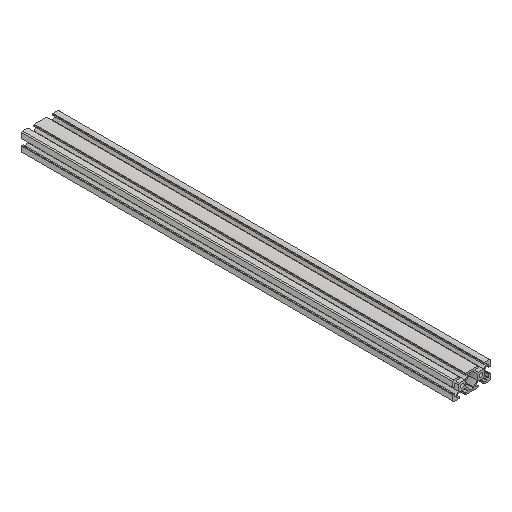
# Autodesk Inventor part: COTS_GENERIC_20x40mm_alu_extrusion_460mm
Saved by Autodesk Inventor 2026.1 (Build 301233000, 233)
## iProperties
Created: 2017-05-24
Part Number: COTS_GENERIC_20x40mm_alu_extrusion_460mm
Material: Ogólny
Document SubType Name: Modeling
Designer: Andrzej
Density: 1 g/cm^3
Appearance: Aluminium - polerowane
Mass: 147.48 g
Surface Area: 1432.83 cm^2
Volume: 147.48 cm^3
Author: Andrzej
Autodesk Inventor part; units mm, degrees
ref_plane "YZ Plane" through (0, 0, 0) normal (1, 0, 0) x (0, 1, 0)
ref_plane "XZ Plane" through (0, 0, 0) normal (0, 1, 0) x (-1, 0, 0)
ref_plane "XY Plane" through (0, 0, 0) normal (0, 0, 1) x (1, 0, 0)
sketch "Szkic1" plane through (0, 0, 0) normal (1, 0, 0) x (0, 1, 0)
  line L0 (23.5169, -0.1319) -> (-36.4831, -0.1319)
  line L1 (-2.0853, 36.7703) -> (-2.0853, -38.5298)
  line L2 (17.9147, 2.8681) -> (15.9147, 2.8681)
  line L3 (17.9147, 2.8681) -> (17.9147, 9.8681)
  line L4 (17.9147, 9.8681) -> (10.9147, 9.8681)
  line L5 (10.9147, 9.8681) -> (10.9147, 7.8681)
  line L6 (15.9147, 2.8681) -> (15.9147, 5.8681)
  line L7 (10.9147, 7.8681) -> (13.9147, 7.8681)
  line L8 (13.9147, 7.8681) -> (13.9147, 6.8681)
  line L9 (15.9147, 5.8681) -> (14.9147, 5.8681)
  line L10 (11.9147, -0.1319) -> (11.9147, 2.8681)
  line L11 (10.9147, 3.8681) -> (4.9147, 3.8681)
  line L12 (3.9147, 2.8681) -> (3.9147, -0.1319)
  line L13 (4.9147, 7.8681) -> (4.9147, 9.8681)
  line L14 (4.9147, 9.8681) -> (-2.0853, 9.8681)
  line L15 (4.9147, 7.8681) -> (1.9147, 7.8681)
  line L16 (1.9147, 7.8681) -> (1.9147, 6.8681)
  line L17 (-0.0853, 7.8681) -> (-0.0853, 6.8681)
  line L18 (-0.0853, 7.8681) -> (-2.0853, 7.8681)
  line L19 (1.9147, 6.8681) -> (4.9147, 3.8681)
  line L20 (1.9147, 6.8681) -> (8.4857, 6.8681) construction
  line L21 (-0.0853, 6.8681) -> (3.9147, 2.8681)
  line L22 (-0.0853, 6.8681) -> (7.9037, 6.8681) construction
  line L23 (14.9147, 5.8681) -> (11.9147, 2.8681)
  line L24 (14.9147, 5.8681) -> (20.5717, 5.8681) construction
  line L25 (13.9147, 6.8681) -> (10.9147, 3.8681)
  line L26 (13.9147, 6.8681) -> (19.5717, 6.8681) construction
  line L27 (17.9147, -3.1319) -> (15.9147, -3.1319)
  line L28 (17.9147, -3.1319) -> (17.9147, -10.1319)
  line L29 (17.9147, -10.1319) -> (10.9147, -10.1319)
  line L30 (10.9147, -10.1319) -> (10.9147, -8.1319)
  line L31 (15.9147, -3.1319) -> (15.9147, -6.1319)
  line L32 (10.9147, -8.1319) -> (13.9147, -8.1319)
  line L33 (13.9147, -8.1319) -> (13.9147, -7.1319)
  line L34 (15.9147, -6.1319) -> (14.9147, -6.1319)
  line L35 (11.9147, -0.1319) -> (11.9147, -3.1319)
  line L36 (10.9147, -4.1319) -> (4.9147, -4.1319)
  line L37 (3.9147, -3.1319) -> (3.9147, -0.1319)
  line L38 (4.9147, -8.1319) -> (4.9147, -10.1319)
  line L39 (4.9147, -10.1319) -> (-2.0853, -10.1319)
  line L40 (4.9147, -8.1319) -> (1.9147, -8.1319)
  line L41 (1.9147, -8.1319) -> (1.9147, -7.1319)
  line L42 (-0.0853, -8.1319) -> (-0.0853, -7.1319)
  line L43 (-0.0853, -8.1319) -> (-2.0853, -8.1319)
  line L44 (1.9147, -7.1319) -> (4.9147, -4.1319)
  line L45 (1.9147, -7.1319) -> (8.4857, -7.1319) construction
  line L46 (-0.0853, -7.1319) -> (3.9147, -3.1319)
  line L47 (-0.0853, -7.1319) -> (7.9037, -7.1319) construction
  line L48 (14.9147, -6.1319) -> (11.9147, -3.1319)
  line L49 (13.9147, -7.1319) -> (10.9147, -4.1319)
  line L50 (13.9147, -7.1319) -> (19.5717, -7.1319) construction
  line L51 (-22.0853, 2.8681) -> (-20.0853, 2.8681)
  line L52 (-22.0853, 2.8681) -> (-22.0853, 9.8681)
  line L53 (-22.0853, 9.8681) -> (-15.0853, 9.8681)
  line L54 (-15.0853, 9.8681) -> (-15.0853, 7.8681)
  line L55 (-20.0853, 2.8681) -> (-20.0853, 5.8681)
  line L56 (-15.0853, 7.8681) -> (-18.0853, 7.8681)
  line L57 (-18.0853, 7.8681) -> (-18.0853, 6.8681)
  line L58 (-20.0853, 5.8681) -> (-19.0853, 5.8681)
  line L59 (-16.0853, -0.1319) -> (-16.0853, 2.8681)
  line L60 (-15.0853, 3.8681) -> (-9.0853, 3.8681)
  line L61 (-8.0853, 2.8681) -> (-8.0853, -0.1319)
  line L62 (-9.0853, 7.8681) -> (-9.0853, 9.8681)
  line L63 (-9.0853, 9.8681) -> (-2.0853, 9.8681)
  line L64 (-9.0853, 7.8681) -> (-6.0853, 7.8681)
  line L65 (-6.0853, 7.8681) -> (-6.0853, 6.8681)
  line L66 (-4.0853, 7.8681) -> (-4.0853, 6.8681)
  line L67 (-4.0853, 7.8681) -> (-2.0853, 7.8681)
  line L68 (-6.0853, 6.8681) -> (-9.0853, 3.8681)
  line L69 (-6.0853, 6.8681) -> (-12.6563, 6.8681) construction
  line L70 (-4.0853, 6.8681) -> (-8.0853, 2.8681)
  line L71 (-4.0853, 6.8681) -> (-12.0743, 6.8681) construction
  line L72 (-19.0853, 5.8681) -> (-16.0853, 2.8681)
  line L73 (-19.0853, 5.8681) -> (-24.7423, 5.8681) construction
  line L74 (-18.0853, 6.8681) -> (-15.0853, 3.8681)
  line L75 (-18.0853, 6.8681) -> (-23.7423, 6.8681) construction
  line L76 (-6.0853, -7.1319) -> (-12.6563, -7.1319) construction
  line L77 (-6.0853, -7.1319) -> (-9.0853, -4.1319)
  line L78 (-4.0853, -7.1319) -> (-12.0743, -7.1319) construction
  line L79 (-4.0853, -8.1319) -> (-4.0853, -7.1319)
  line L80 (-4.0853, -7.1319) -> (-8.0853, -3.1319)
  line L81 (-6.0853, -8.1319) -> (-6.0853, -7.1319)
  line L82 (-9.0853, -8.1319) -> (-6.0853, -8.1319)
  line L83 (-4.0853, -8.1319) -> (-2.0853, -8.1319)
  line L84 (-15.0853, -10.1319) -> (-15.0853, -8.1319)
  line L85 (-9.0853, -10.1319) -> (-2.0853, -10.1319)
  line L86 (-9.0853, -8.1319) -> (-9.0853, -10.1319)
  line L87 (-15.0853, -4.1319) -> (-9.0853, -4.1319)
  line L88 (-8.0853, -3.1319) -> (-8.0853, -0.1319)
  line L89 (-22.0853, -3.1319) -> (-20.0853, -3.1319)
  line L90 (-22.0853, -3.1319) -> (-22.0853, -10.1319)
  line L91 (-22.0853, -10.1319) -> (-15.0853, -10.1319)
  line L92 (-20.0853, -3.1319) -> (-20.0853, -6.1319)
  line L93 (-15.0853, -8.1319) -> (-18.0853, -8.1319)
  line L94 (-18.0853, -8.1319) -> (-18.0853, -7.1319)
  line L95 (-20.0853, -6.1319) -> (-19.0853, -6.1319)
  line L96 (-18.0853, -7.1319) -> (-15.0853, -4.1319)
  line L97 (-19.0853, -6.1319) -> (-16.0853, -3.1319)
  line L98 (-18.0853, -7.1319) -> (-23.7423, -7.1319) construction
  line L99 (-16.0853, -0.1319) -> (-16.0853, -3.1319)
  point P0 (0, 0)
  point P1 (0, -0.2637)
  point P2 (-4.1707, 0)
  point P3 (-4.1707, -0.2637)
  dimension "d1" = 2
  dimension "d2" = 3
  dimension "d3" = 7
  dimension "d4" = 7
  dimension "d5" = 2
  dimension "d6" = 3
  dimension "d7" = 3
  dimension "d8" = 1
  dimension "d9" = 1
  dimension "d12" = 6
  dimension "d13" = 2
  dimension "d14" = 7
  dimension "d15" = 6
  dimension "d16" = 3
  dimension "d17" = 1
  dimension "d18" = 1
  dimension "d19" = 2
  dimension "d20" = 8
  dimension "d22" = 45
  dimension "d24" = 45
  dimension "d26" = 135
  dimension "d28" = 135
  dimension "d29" = 6
  dimension "d30" = 4
  dimension "d31" = 3
  dimension "d32" = 3
  dimension "d33" = 8
  dimension "d34" = 1
  constraints: 200 end point, 74 symmetric about line, 9 horizontal, 9 vertical, 5 perpendicular, 4 point on line
  measures "d1" distance of L2.start L2.end
  measures "d2" distance between parallel lines of L0 L2
  measures "d3" distance of L2.start L3.end
  measures "d4" distance of L3.end L4.end
  measures "d5" distance of L4.end L5.end
  measures "d6" distance of L2.end L6.end
  measures "d7" distance of L5.end L7.end
  measures "d8" distance of L7.end L8.end
  measures "d9" distance of L6.end L9.end
  measures "d12" distance between parallel lines of L3 L10
  measures "d13" distance of L13.start L13.end
  measures "d14" distance of L13.end L14.end
  measures "d15" distance between parallel lines of L5 L13
  measures "d16" distance of L13.start L15.end
  measures "d17" distance of L15.end L16.end
  measures "d18" distance of L17.start L17.end
  measures "d19" distance between parallel lines of L16 L17
  measures "d20" distance between parallel lines of L0 L15
  measures "d22" angle of L19 L20
  measures "d24" angle of L21 L22
  measures "d26" angle of L23 L24
  measures "d28" angle of L25 L26
  measures "d29" distance of L11.start L11.end
  measures "d30" distance between parallel lines of L0 L11
  measures "d31" distance of L10.start L10.end
  measures "d32" distance of L12.start L12.end
  measures "d33" distance between parallel lines of L10 L12
  measures "d34" distance from line of L10 L11.start
extrude "Wyciągnięcie proste1" add sketch "Szkic1" along normal blind 460 contours L35 L48 L34 L31 L27 L28 L29 L30 L32 L33 L49 L36 L44 L41 L40 L38 L39 L1 L43 L42 L46 L37 L0 | L0 L12 L21 L17 L18 L1 L14 L13 L15 L16 L19 L11 L25 L8 L7 L5 L4 L3 L2 L6 L9 L23 L10 | L88 L80 L79 L83 L1 L85 L86 L82 L81 L77 L87 L96 L94 L93 L84 L91 L90 L89 L92 L95 L97 L99 L0 | L0 L59 L72 L58 L55 L51 L52 L53 L54 L56 L57 L74 L60 L68 L65 L64 L62 L63 L1 L67 L66 L70 L61
sketch "Szkic2" plane through (460, 0, 0) normal (1, 0, 0) x (0, 0, -1)
  line L0 (-7.8681, -4.0853) -> (-7.8681, -0.0853) projected
  line L1 (-7.8681, -0.0853) -> (-6.8681, -0.0853) projected
  line L2 (-6.8681, -0.0853) -> (-2.8681, 3.9147) projected
  line L3 (-2.8681, 3.9147) -> (3.1319, 3.9147) projected
  line L4 (3.1319, 3.9147) -> (7.1319, -0.0853) projected
  line L5 (7.1319, -0.0853) -> (8.1319, -0.0853) projected
  line L6 (8.1319, -0.0853) -> (8.1319, -4.0853) projected
  line L7 (8.1319, -4.0853) -> (7.1319, -4.0853) projected
  line L8 (7.1319, -4.0853) -> (3.1319, -8.0853) projected
  line L9 (3.1319, -8.0853) -> (-2.8681, -8.0853) projected
  line L10 (-2.8681, -8.0853) -> (-6.8681, -4.0853) projected
  line L11 (-6.8681, -4.0853) -> (-7.8681, -4.0853) projected
  line L12 (-9.8681, 4.9147) -> (-9.8681, -9.0853) projected
  line L13 (-9.8681, -9.0853) -> (-7.8681, -9.0853) projected
  line L14 (-7.8681, -9.0853) -> (-7.8681, -6.0853) projected
  line L15 (-7.8681, -6.0853) -> (-6.8681, -6.0853) projected
  line L16 (-6.8681, -6.0853) -> (-3.8681, -9.0853) projected
  line L17 (-3.8681, -9.0853) -> (-3.8681, -15.0853) projected
  line L18 (-3.8681, -15.0853) -> (-6.8681, -18.0853) projected
  line L19 (-6.8681, -18.0853) -> (-7.8681, -18.0853) projected
  line L20 (-7.8681, -18.0853) -> (-7.8681, -15.0853) projected
  line L21 (-7.8681, -15.0853) -> (-9.8681, -15.0853) projected
  line L22 (-9.8681, -15.0853) -> (-9.8681, -22.0853) projected
  line L23 (-9.8681, -22.0853) -> (-2.8681, -22.0853) projected
  line L24 (-2.8681, -22.0853) -> (-2.8681, -20.0853) projected
  line L25 (-2.8681, -20.0853) -> (-5.8681, -20.0853) projected
  line L26 (-5.8681, -20.0853) -> (-5.8681, -19.0853) projected
  line L27 (-5.8681, -19.0853) -> (-2.8681, -16.0853) projected
  line L28 (-2.8681, -16.0853) -> (3.1319, -16.0853) projected
  line L29 (3.1319, -16.0853) -> (6.1319, -19.0853) projected
  line L30 (6.1319, -19.0853) -> (6.1319, -20.0853) projected
  line L31 (6.1319, -20.0853) -> (3.1319, -20.0853) projected
  line L32 (3.1319, -20.0853) -> (3.1319, -22.0853) projected
  line L33 (3.1319, -22.0853) -> (10.1319, -22.0853) projected
  line L34 (10.1319, -22.0853) -> (10.1319, -15.0853) projected
  line L35 (10.1319, -15.0853) -> (8.1319, -15.0853) projected
  line L36 (8.1319, -15.0853) -> (8.1319, -18.0853) projected
  line L37 (8.1319, -18.0853) -> (7.1319, -18.0853) projected
  line L38 (7.1319, -18.0853) -> (4.1319, -15.0853) projected
  line L39 (4.1319, -15.0853) -> (4.1319, -9.0853) projected
  line L40 (4.1319, -9.0853) -> (7.1319, -6.0853) projected
  line L41 (7.1319, -6.0853) -> (8.1319, -6.0853) projected
  line L42 (8.1319, -6.0853) -> (8.1319, -9.0853) projected
  line L43 (8.1319, -9.0853) -> (10.1319, -9.0853) projected
  line L44 (10.1319, -9.0853) -> (10.1319, 4.9147) projected
  line L45 (10.1319, 4.9147) -> (8.1319, 4.9147) projected
  line L46 (8.1319, 4.9147) -> (8.1319, 1.9147) projected
  line L47 (8.1319, 1.9147) -> (7.1319, 1.9147) projected
  line L48 (7.1319, 1.9147) -> (4.1319, 4.9147) projected
  line L49 (4.1319, 4.9147) -> (4.1319, 10.9147) projected
  line L50 (4.1319, 10.9147) -> (7.1319, 13.9147) projected
  line L51 (7.1319, 13.9147) -> (8.1319, 13.9147) projected
  line L52 (8.1319, 13.9147) -> (8.1319, 10.9147) projected
  line L53 (8.1319, 10.9147) -> (10.1319, 10.9147) projected
  line L54 (10.1319, 10.9147) -> (10.1319, 17.9147) projected
  line L55 (10.1319, 17.9147) -> (3.1319, 17.9147) projected
  line L56 (3.1319, 17.9147) -> (3.1319, 15.9147) projected
  line L57 (3.1319, 15.9147) -> (6.1319, 15.9147) projected
  line L58 (6.1319, 15.9147) -> (6.1319, 14.9147) projected
  line L59 (6.1319, 14.9147) -> (3.1319, 11.9147) projected
  line L60 (3.1319, 11.9147) -> (-2.8681, 11.9147) projected
  line L61 (-2.8681, 11.9147) -> (-5.8681, 14.9147) projected
  line L62 (-5.8681, 14.9147) -> (-5.8681, 15.9147) projected
  line L63 (-5.8681, 15.9147) -> (-2.8681, 15.9147) projected
  line L64 (-2.8681, 15.9147) -> (-2.8681, 17.9147) projected
  line L65 (-2.8681, 17.9147) -> (-9.8681, 17.9147) projected
  line L66 (-9.8681, 17.9147) -> (-9.8681, 10.9147) projected
  line L67 (-9.8681, 10.9147) -> (-7.8681, 10.9147) projected
  line L68 (-7.8681, 10.9147) -> (-7.8681, 13.9147) projected
  line L69 (-7.8681, 13.9147) -> (-6.8681, 13.9147) projected
  line L70 (-6.8681, 13.9147) -> (-3.8681, 10.9147) projected
  line L71 (-3.8681, 10.9147) -> (-3.8681, 4.9147) projected
  line L72 (-3.8681, 4.9147) -> (-6.8681, 1.9147) projected
  line L73 (-6.8681, 1.9147) -> (-7.8681, 1.9147) projected
  line L74 (-7.8681, 1.9147) -> (-7.8681, 4.9147) projected
  line L75 (-7.8681, 4.9147) -> (-9.8681, 4.9147) projected
  point P0 (0, 0)
  point P1 (0.1319, 7.9147)
  point P2 (0.1319, -12.0853)
  dimension "d37" = 4
  dimension "d38" = 4
  dimension "d39" = 4
  dimension "d40" = 4
  measures "d37" distance from line of L60 point (0.132, 7.915)
  measures "d38" distance from line of L49 point (0.132, 7.915)
  measures "d39" distance from line of L9 point (0.132, -12.085)
  measures "d40" distance from line of L39 point (0.132, -12.085)
hole "Otwór1" at (460, 7.9147, -0.1319) at (460, -12.0853, -0.1319) direction (-1, 0, 0) diameter 4.2 end through all
fillet "Zaokrąglenie1" radius 1 4 edges at (230, 17.9147, -10.1319) (230, 17.9147, 9.8681) (230, -22.0853, -10.1319) (230, -22.0853, 9.8681)
fillet "Zaokrąglenie2" radius 0.4 24 edges at (230, 4.9147, -10.1319) (230, 4.9147, -8.1319) (230, 10.9147, -10.1319) (230, 10.9147, -8.1319) (230, 17.9147, -3.1319) (230, 15.9147, -3.1319) (230, 10.9147, 9.8681) (230, 17.9147, 2.8681) (230, 10.9147, 7.8681) (230, 15.9147, 2.8681) (230, 4.9147, 7.8681) (230, 4.9147, 9.8681) (230, -9.0853, 7.8681) (230, -9.0853, 9.8681) (230, -15.0853, 7.8681) (230, -15.0853, 9.8681) (230, -9.0853, -10.1319) (230, -9.0853, -8.1319) (230, -15.0853, -10.1319) (230, -15.0853, -8.1319) (230, -20.0853, -3.1319) (230, -22.0853, -3.1319) (230, -22.0853, 2.8681) (230, -20.0853, 2.8681)
